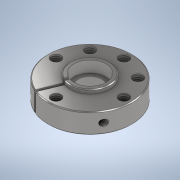
# Autodesk Inventor part: ClampHorn
Saved by Autodesk Inventor 2020 (Build 240168000, 168)
## iProperties
Part Number: ClampHorn
Material: 一般
Document SubType Name: Modeling
Designer: MasatoKubotera
Density: 1 g/cm^3
Appearance: 半つや出し
Catalog Web Link: https://kondo-robot.com/product/02031
Description: ReadyMade
Author: MasatoKubotera
Autodesk Inventor part; units mm, degrees
ref_plane "YZ Plane" through (0, 0, 0) normal (1, 0, 0) x (0, 1, 0)
ref_plane "XY Plane" through (0, 0, 0) normal (0, 0, 1) x (1, 0, 0)
sketch "スケッチ1" plane through (0, 0, 0) normal (0, 1, 0) x (-1, 0, 0)
  line L0 (-3.05, 0) -> (-3.05, 1.5)
  line L1 (-3.05, 1.5) -> (-3, 1.5)
  line L2 (-3, 1.5) -> (-3, 4.5)
  line L3 (-3, 4.5) -> (-4, 4.5)
  line L4 (-4, 7.3) -> (-5, 7.3)
  line L5 (-5, 7.3) -> (-5, 6.3)
  line L6 (-5, 6.3) -> (-10.5, 6.3)
  line L7 (-10.5, 6.3) -> (-10.5, 1.3)
  line L8 (-10.5, 1.3) -> (-6.5, 1.3)
  line L9 (-6.5, 1.3) -> (-6.5, 2.2)
  line L10 (-6.5, 2.2) -> (-5, 2.2)
  line L11 (-5, 2.2) -> (-5, 1.7)
  line L12 (-5, 1.7) -> (-4, 1.7)
  line L13 (-4, 1.7) -> (-4, 0)
  line L14 (-4, 0) -> (-3.05, 0)
  line L15 (0, -1.46) -> (0, 8.76) projected
  line L16 (-4, 7.3) -> (-4, 4.5)
  line L17 (2.1, 0) -> (-12.6, 0) projected
  point P0 (0, 0)
  dimension "d0" = 6.1
  dimension "d1" = 8
  dimension "d2" = 10
  dimension "d3" = 13
  dimension "d4" = 21
  dimension "d5" = 6
  dimension "d6" = 8
  dimension "d7" = 10
  dimension "d8" = 5
  dimension "d9" = 1
  dimension "d10" = 2.8
  dimension "d11" = 1.5
  dimension "d12" = 3
  dimension "d13" = 1.7
  dimension "d14" = 0.5
  dimension "d15" = 0.9
  constraints: 32 end point, 13 perpendicular, 1 collinear, 1 vertical
  measures "d0" diameter of L0 L15
  measures "d1" diameter of L13 L15
  measures "d2" diameter of L11 L15
  measures "d3" diameter of L9 L15
  measures "d4" diameter of L7 L15
  measures "d5" diameter of L2 L15
  measures "d6" diameter of L16 L15
  measures "d7" diameter of L5 L15
  measures "d8" distance of L6.end L7.end
  measures "d9" distance of L4.end L5.end
  measures "d10" distance of L4.start L3.end
  measures "d11" distance of L0.start L0.end
  measures "d12" distance of L1.end L2.end
  measures "d13" distance of L12.end L13.end
  measures "d14" distance of L10.end L11.end
  measures "d15" distance of L8.end L9.end
revolve "回転1" add sketch "スケッチ1" angle 360 about axis through (0, 0, -10) along (0, 0, 1)
sketch "スケッチ2" plane through (0, 0, 6.3) normal (0, 0, 1) x (1, 0, 0)
  line L0 (-14.7, 0) -> (14.7, 0) projected
  line L1 (0, 0) -> (9.7007, -4.0182) construction
  circle A0 centre (0, 0) radius 10.5 projected
  line L2 (9.8116, -3.7394) -> (2.8726, -0.8651)
  circle A1 centre (0, 0) radius 3 projected
  line L3 (9.582, -4.2937) -> (2.6429, -1.4195)
  line L4 (5.5, 8.9443) -> (5.5, 0) construction
  line L5 (5.5, 0) -> (5.5, -8.9443) construction
  line L6 (5.5, -7.245) -> (7.6, -7.245) construction
  point P0 (-8.5, 0)
  point P1 (2.6429, -1.4195)
  dimension "d17" = 8.5
  dimension "d29" = 0.6
  dimension "d30" = 22.5
  dimension "d41" = 5.5
  dimension "d42" = 8.9443
  dimension "d62" = 4.2
  dimension "d63" = 1.6993
  constraints: 12 end point, 5 point on circle, 3 point on line, 2 perpendicular, 2 symmetric about line, 1 horizontal, 1 parallel, 2 other
  measures "d17" distance of L1.start point (-8.5, 0)
  measures "d29" distance of L2.start L3.start
  measures "d30" angle of L0 L1
  measures "d41" horizontal distance of L1.start L4.start
  measures "d42" distance of L4.end L5.end
  measures "d62" diameter of L6.end L5
  measures "d63" vertical distance of L5.end L6.end
hole "穴1" at (-8.5, 0, 6.3) direction (0, 0, -1) diameter 2.459 end through all thread size "M3x0.5" class "6H" standard "ISO Metric profile"
pattern_circular "円形状パターン1" count 8 over 360 about axis through (0, 0, -10) along (0, 0, 1) of "穴1" skipped copies 4 6
extrude "押し出し1" cut sketch "スケッチ2" against normal through all both and the other way through all contours L2 A0 L3 A1
ref_plane "作業平面1" through (0, -8.9443, 0) normal (0, 1, 0) x (-1, 0, 0)
sketch "スケッチ3" plane through (0, -8.9443, 0) normal (0, 1, 0) x (-1, 0, 0)
  circle A0 centre (-5.5, 3.8) radius 2.1
  line L0 (-5.5, 6.3) -> (-5.5, 1.3) construction
  line L1 (10.5, 1.3) -> (-10.5, 1.3) projected
  circle A1 centre (-5.5, 3.8) radius 1.15
  point P0 (0, 0)
  point P1 (-9.8116, 1.3)
  point P2 (-9.582, 1.3)
  dimension "d44" = 4.2
  dimension "d45" = 2.3
  constraints: 3 coincident, 2 centre point, 2 end point, 1 midpoint, 1 point on line, 1 vertical
  measures "d44" diameter of A0
  measures "d45" diameter of A1
hole "穴3" at (5.5, -8.9443, 3.8) direction (0, 1, 0) diameter 1.567 end through all thread size "M2x0.4" class "6H" standard "ISO Metric profile"
extrude "押し出し2" cut sketch "スケッチ3" along normal up to surface (8.9443 mm away) contours A1
extrude "押し出し3" cut sketch "スケッチ3" along normal blind 3.4443
extrude "押し出し4" cut sketch "スケッチ3" against normal through all contours A0 | A1
chamfer "面取り1" distance 0.2 angle 45 4 edges at (-4.6194, 1.9134, 7.3) (-9.7007, 4.0182, 6.3) (-9.7007, 4.0182, 1.3) (-3.6955, 1.5307, 0)
equation "\"d23\" = d2 + d8"
equation "\"d43\" = -d42"
